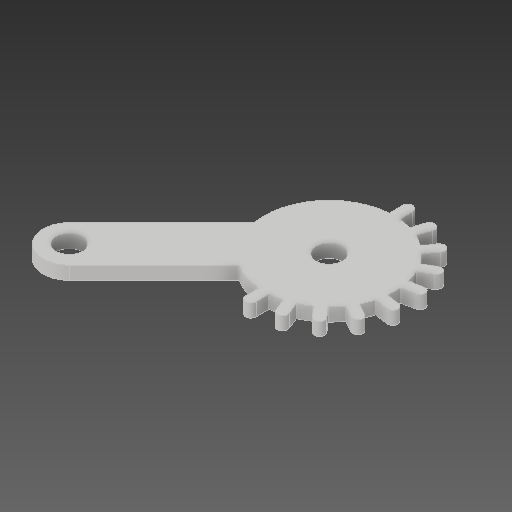
# Autodesk Inventor part: gerigi
Saved by Autodesk Inventor 2019 (Build 230136000, 136)
## iProperties
Created: 2016-12-01
Part Number: gerigi
Material: Generic
Document SubType Name: Modeling
Designer: MuhammadArdian
Density: 1 g/cm^3
Appearance: Default
Author: MuhammadArdian
Autodesk Inventor part; units mm, degrees
ref_plane "YZ Plane" through (0, 0, 0) normal (1, 0, 0) x (0, 1, 0)
ref_plane "XZ Plane" through (0, 0, 0) normal (0, 1, 0) x (-1, 0, 0)
ref_plane "XY Plane" through (0, 0, 0) normal (0, 0, 1) x (1, 0, 0)
sketch "Sketch1" plane through (0, 0, 0) normal (0, 1, 0) x (-1, 0, 0)
  line L0 (-2.1276, -24.9093) -> (-2.0134, -30.0178)
  line L1 (1.9856, -29.9284) -> (1.8739, -24.9297)
  arc A0 (-2.0134, -30.0178) -> (1.9856, -29.9284) centre (-0.0139, -29.9731) ccw
  arc A1 (-12.1587, -27.5189) -> (-8.3703, -28.8026) centre (-10.2645, -28.1608) ccw
  line L2 (-8.3703, -28.8026) -> (-6.7656, -24.0671)
  line L3 (-10.5187, -22.6794) -> (-12.1587, -27.5189)
  arc A2 (-20.8374, -21.7008) -> (-17.7166, -24.2028) centre (-19.277, -22.9518) ccw
  line L4 (-17.7166, -24.2028) -> (-14.589, -20.3017)
  line L5 (-17.6412, -17.7141) -> (-20.8374, -21.7008)
  arc A3 (-27.0029, -13.2653) -> (-24.926, -16.6838) centre (-25.9644, -14.9745) ccw
  line L6 (-24.926, -16.6838) -> (-20.6528, -14.0877)
  line L7 (-22.6359, -10.6121) -> (-27.0029, -13.2653)
  arc A4 (-29.9114, -3.2297) -> (-29.1289, -7.1525) centre (-29.5202, -5.1911) ccw
  line L8 (-29.1289, -7.1525) -> (-24.2255, -6.1744)
  line L9 (-24.9003, -2.2302) -> (-29.9114, -3.2297)
  arc A5 (-29.2121, 7.1953) -> (-29.8185, 3.2416) centre (-29.5153, 5.2185) ccw
  line L10 (-29.8185, 3.2416) -> (-24.8763, 2.4836)
  line L11 (-24.1614, 6.4207) -> (-29.2121, 7.1953)
  arc A6 (-24.9895, 16.7526) -> (-26.9116, 13.2446) centre (-25.9505, 14.9986) ccw
  line L12 (-26.9116, 13.2446) -> (-22.5267, 10.842)
  line L13 (-20.5083, 14.2972) -> (-24.9895, 16.7526)
  arc A7 (-17.7527, 24.2892) -> (-20.7587, 21.6502) centre (-19.2557, 22.9697) ccw
  line L14 (-20.7587, 21.6502) -> (-17.46, 17.8927)
  line L15 (-14.3816, 20.4492) -> (-17.7527, 24.2892)
  arc A8 (-8.3747, 28.8961) -> (-12.102, 27.4444) centre (-10.2384, 28.1703) ccw
  line L16 (-12.102, 27.4444) -> (-10.2873, 22.7853)
  line L17 (-6.5202, 24.1348) -> (-8.3747, 28.8961)
  arc A9 (2.0134, 30.0178) -> (-1.9856, 29.9284) centre (0.0139, 29.9731) ccw
  line L18 (-1.9856, 29.9284) -> (-1.8739, 24.9297)
  line L19 (2.1276, 24.9093) -> (2.0134, 30.0178)
  arc A10 (1.8739, -24.9297) -> (24.6616, 4.0993) centre (0, 0) ccw
  circle A11 centre (52.9459, 46.5257) radius 5
  line L20 (45.8748, 53.5968) -> (13.3899, 21.1118)
  line L21 (24.6616, 4.0993) -> (60.017, 39.4546)
  arc A12 (60.017, 39.4546) -> (45.8748, 53.5968) centre (52.9459, 46.5257) ccw
  arc A13 (13.3899, 21.1118) -> (2.1276, 24.9093) centre (0, 0) ccw
  arc A14 (-1.8739, 24.9297) -> (-6.5202, 24.1348) centre (0, 0) ccw
  arc A15 (-10.2873, 22.7853) -> (-14.3816, 20.4492) centre (0, 0) ccw
  arc A16 (-17.46, 17.8927) -> (-20.5083, 14.2972) centre (0, 0) ccw
  arc A17 (-22.5267, 10.842) -> (-24.1614, 6.4207) centre (0, 0) ccw
  arc A18 (-24.8763, 2.4836) -> (-24.9003, -2.2302) centre (0, 0) ccw
  arc A19 (-24.2255, -6.1744) -> (-22.6359, -10.6121) centre (0, 0) ccw
  arc A20 (-20.6528, -14.0877) -> (-17.6412, -17.7141) centre (0, 0) ccw
  arc A21 (-14.589, -20.3017) -> (-10.5187, -22.6794) centre (0, 0) ccw
  arc A22 (-6.7656, -24.0671) -> (-2.1276, -24.9093) centre (0, 0) ccw
  circle A23 centre (0, 0) radius 5
  point P0 (28.2843, 28.2843)
  dimension "d9" = 180
  dimension "d17" = 10
  dimension "d18" = 10
  dimension "d19" = 20
  dimension "d20" = 25
  dimension "d21" = 5
  dimension "d22" = 2
  dimension "d23" = 50
  constraints: 44 end point, 44 point on circle, 24 centre point, 4 tangent, 3 coincident, 2 parallel, 81 other
  measures "d17" diameter of A11
  measures "d18" diameter of A23
  measures "d19" distance between parallel lines of L20 L21
  measures "d20" radius of A14
  measures "d21" distance of L1.start L1.end
  measures "d22" radius of A9
  measures "d23" distance of L21.start L21.end
extrude "Extrusion1" add sketch "Sketch1" along normal blind 5
body "Solid1"
